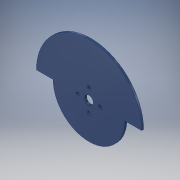
# Autodesk Inventor part: PixyCamGimbal Base
Saved by Autodesk Inventor 2017 (Build 210142000, 142)
## iProperties
Created: 2016-12-06
Part Number: PixyCamGimbal Base
Material: Generic
Document SubType Name: Modeling
Designer: PLTW
Density: 1 g/cm^3
Appearance: Flaked Satin - Blue
Author: PLTW
Autodesk Inventor part; units mm, degrees
ref_plane "YZ Plane" through (0, 0, 0) normal (1, 0, 0) x (0, 1, 0)
ref_plane "XZ Plane" through (0, 0, 0) normal (0, 1, 0) x (-1, 0, 0)
ref_plane "XY Plane" through (0, 0, 0) normal (0, 0, 1) x (1, 0, 0)
sketch "Sketch1" plane through (0, 0, 0) normal (0, 0, 1) x (1, 0, 0)
  circle A0 centre (0, 0) radius 3.556
  circle A1 centre (0, 9.144) radius 1.27
  circle A2 centre (-9.144, 0) radius 1.27
  circle A3 centre (0, -9.144) radius 1.27
  circle A4 centre (9.144, 0) radius 1.27
  arc A5 (43.18, 0) -> (-43.18, 0) centre (0, 0) ccw
  arc A6 (-29.464, 0) -> (29.464, 0) centre (0, 0) ccw
  line L0 (-43.18, 0) -> (-29.464, 0)
  line L1 (29.464, 0) -> (43.18, 0)
  circle A7 centre (0, 35.56) radius 0.127
  circle A8 centre (0, -22.098) radius 0.127
  circle A9 centre (-34.798, 7.366) radius 0.127
  circle A10 centre (34.798, 7.366) radius 0.127
  dimension "d0" = 7.112
  dimension "d1" = 2.54
  dimension "d2" = 9.144
  dimension "d5" = 360
  dimension "d7" = 43.18
  dimension "d8" = 29.464
  dimension "d9" = 35.56
  dimension "d10" = 34.798
  dimension "d11" = 34.798
  dimension "d12" = 22.098
  dimension "d13" = 0.254
  dimension "d14" = 7.366
  constraints: 11 centre point, 5 horizontal alignment, 4 end point, 4 point on circle, 3 equal radius, 3 vertical alignment, 2 concentric, 1 coincident, 1 collinear, 1 horizontal, 9 other
  measures "d0" diameter of A0
  measures "d1" diameter of A1
  measures "d2" distance of point (0, 0) A1.centre
  measures "d7" radius of A5
  measures "d8" radius of A6
  measures "d9" distance of point (0, 0) A7.centre
  measures "d10" horizontal distance of point (0, 0) A9.centre
  measures "d11" horizontal distance of A10.centre point (0, 0)
  measures "d12" distance of A8.centre A0.centre
  measures "d13" diameter of A7
  measures "d14" distance from line of L0 A9.centre
extrude "Extrusion1" add sketch "Sketch1" along normal blind 1.5875
equation "\"d11\" = d10"
body "Solid1"
